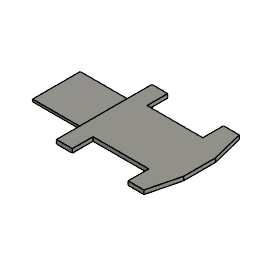
BottomBack (Autodesk Fusion 360 design; units mm, degrees)
part number: 2026-01-06-13-16-38-039
Autodesk Fusion 360 part; units mm, degrees
sketch "Bottom back base" plane through (0, 0, 0) normal (0, 0, 1) x (1, 0, 0)
  line L0 (-60, 60) -> (-60, -60)
  line L1 (60, -20) -> (60, 20)
  line L2 (-60, 0) -> (-57.5, 0) construction
  line L3 (-57.5, -60) -> (-57.5, -6) construction
  line L4 (-57.5, -6) -> (12.5, -6) construction
  line L5 (12.5, -6) -> (12.5, -34) construction
  line L6 (12.5, -34) -> (30, -34)
  line L7 (30, -34) -> (12.5, -34)
  line L8 (12.5, -34) -> (-40, -34)
  line L9 (-40, -34) -> (-40, -60)
  line L10 (30, -34) -> (30, -60)
  line L11 (-40, 34) -> (-40, 60)
  line L12 (12.5, 34) -> (-40, 34)
  line L13 (12.5, 34) -> (30, 34)
  line L14 (30, 34) -> (30, 60)
  line L15 (50, -60) -> (60, -20)
  line L16 (50, 60) -> (60, 20)
  line L17 (50, 60) -> (30, 60)
  line L18 (-40, 60) -> (-60, 60)
  line L19 (-60, -60) -> (-40, -60)
  line L20 (30, -60) -> (50, -60)
  point P0 (60, 60)
  point P1 (60, -60)
  dimension "d1" = 120
  dimension "d2" = 120
  dimension "d3" = 2.5
  dimension "d4" = 54
  dimension "d5" = 70
  dimension "d6" = 28
  dimension "d8" = 70
  dimension "d9" = 10
  dimension "d10" = 40
  dimension "d11" = 10
  dimension "d12" = 40
  constraint horizontal L17
  constraint perpendicular L0 L17
  constraint parallel L17 L19
  constraint parallel L0 L1
  constraint midpoint L0 L2.start
  constraint perpendicular L0 L2
  constraint coincident L3.start L19
  constraint perpendicular L3 L19
  constraint perpendicular L3 L4
  constraint perpendicular L4 L5
  constraint perpendicular L5 L6
  constraint perpendicular L5 L8
  constraint perpendicular L9 L19
  constraint coincident L10.end L19
  constraint perpendicular L10 L19
  constraint symmetric L2 L5.end L12.start
  constraint symmetric L2 L6.end L13.end
  constraint symmetric L2 L8.end L11.start
  constraint symmetric L2 L9.end L11.end
  constraint symmetric L2 L10.end L14.end
  constraint coincident P1 L19
  constraint coincident P1 L1
  constraint coincident P0 L17
  constraint coincident P0 L1
  constraint collinear L17 L18
  constraint collinear L19 L20
  measures "d1" distance of L0.start L0.end
  measures "d2" distance of P0 L0.start
  measures "d3" distance of L2.start L2.end
  measures "d4" distance of L3.start L3.end
  measures "d5" distance of L3.end L4.end
  measures "d6" distance of L4.end L5.end
  measures "d8" distance of L6.end L8.end
  measures "d9" distance of P1 L15.start
  measures "d10" distance of P1 L1.start
  measures "d11" distance of P0 L16.start
  measures "d12" distance of P0 L1.end
extrude "Bottom back height" add sketch "Bottom back base" along normal blind 5
sketch "Connector" plane through (-60, 0, 0) normal (-1, 0, 0) x (0, -1, 0)
  line L0 (-60, 0) -> (60, 0)
  line L1 (60, 0) -> (60, 5)
  line L2 (60, 5) -> (-60, 5)
  line L3 (-60, 5) -> (-60, 0)
  line L4 (0, 0) -> (0, 5) construction
  line L5 (30, 4) -> (-30, 4)
  line L6 (-30, 4) -> (-30, 1)
  line L7 (-30, 1) -> (30, 1)
  line L8 (30, 1) -> (30, 4)
  line L9 (30, 4) -> (-30, 1) construction
  line L10 (-30, 4) -> (30, 1) construction
  point P0 (0, 2.5)
  dimension "d15" = 3
  dimension "d16" = 60
  constraint coincident L4.start origin
  constraint midpoint L2 L4.end
  constraint horizontal L5
  constraint perpendicular L5 L6
  constraint parallel L5 L7
  constraint parallel L6 L8
  constraint coincident L9 P0
  constraint coincident L10 P0
  constraint midpoint L4 P0
  measures "d15" distance of L5.end L6.end
  measures "d16" distance of L5.start L5.end
extrude "Connector width" add sketch "Connector" along normal blind 60 contours L5 L6 L7 L8
equation "d6 = 54 mm - 26 mm"
named bodies: "Bottom back"
